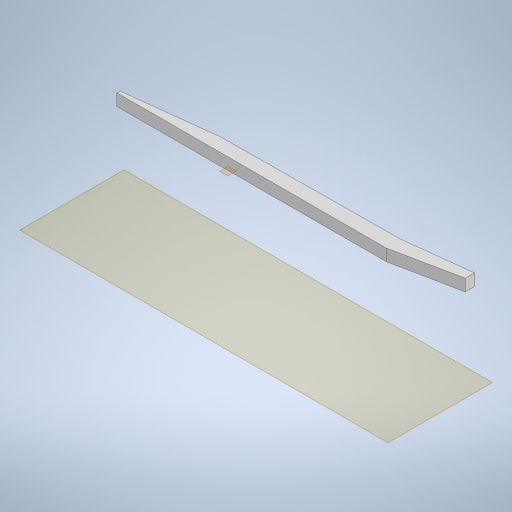
# Autodesk Inventor part: Friend_sideskirt_collision
Saved by Autodesk Inventor 2024 (Build 280153000, 153)
## iProperties
Created: 2026-05-25
Part Number: Friend_sideskirt_collision
Material: Generic
Document SubType Name: Modeling
Designer: warny
Density: 1 g/cm^3
Appearance: Default
Author: warny
Autodesk Inventor part; units mm, degrees
ref_plane "YZ Plane" through (0, 0, 0) normal (1, 0, 0) x (0, 1, 0)
ref_plane "XY Plane" through (0, 0, 0) normal (0, 0, 1) x (1, 0, 0)
ref_plane "Work Plane1" through (0, 193, 0) normal (0, 1, 0) x (-1, 0, 0)
sketch "Sketch1" plane through (0, 193, 0) normal (0, 1, 0) x (-1, 0, 0)
  line L0 (0, -83.592) -> (0, 13.932) construction
  line L1 (438.46, 0) -> (-674.96, 0) construction
  line L2 (279.4, -15.35) -> (278.2, -22.85)
  line L3 (278.2, -22.85) -> (65, -47.86)
  line L4 (65, -47.86) -> (-358.9, -51.36)
  line L5 (-358.9, -51.36) -> (-515.9, -69.66)
  line L6 (-515.9, -69.66) -> (-515.9, -47.66)
  line L7 (-515.9, -47.66) -> (-359.9, -15.93)
  line L8 (-359.9, -15.93) -> (279.4, -15.35)
  point P0 (0, 0)
  dimension "d1" = 22.85
  dimension "d2" = 47.86
  dimension "d3" = 15.35
  dimension "d4" = 279.4
  dimension "d5" = 278.2
  dimension "d6" = 65
  dimension "d7" = 51.36
  dimension "d8" = 69.66
  dimension "d9" = 47.66
  dimension "d10" = 15.93
  dimension "d11" = 515.9
  dimension "d12" = 515.9
  dimension "d13" = 358.9
  dimension "d14" = 359.9
  constraints: 14 end point
  measures "d1" distance from line of L1 L2.end
  measures "d2" distance from line of L1 L3.end
  measures "d3" distance from line of L1 L2.start
  measures "d4" distance from line of L0 L2.start
  measures "d5" distance from line of L0 L2.end
  measures "d6" distance from line of L0 L3.end
  measures "d7" distance from line of L1 L4.end
  measures "d8" distance from line of L1 L5.end
  measures "d9" distance from line of L1 L6.end
  measures "d10" distance from line of L1 L7.end
  measures "d11" distance from line of L0 L5.end
  measures "d12" distance from line of L0 L6.end
  measures "d13" distance from line of L0 L4.end
  measures "d14" distance from line of L0 L7.end
extrude "Extrusion1" add sketch "Sketch1" along normal mid plane 28
body "Solid1"
